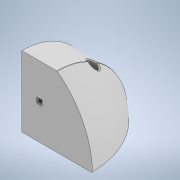
# Autodesk Inventor part: 3DPrintShape
Saved by Autodesk Inventor 2022 (Build 260153000, 153)
## iProperties
Created: 2022-04-20
Part Number: 3DPrintShape
Material: Generic
Document SubType Name: Modeling
Designer: Bruger
Density: 1 g/cm^3
Appearance: Default
Author: Bruger
Autodesk Inventor part; units mm, degrees
ref_plane "YZ Plane" through (0, 0, 0) normal (1, 0, 0) x (0, 1, 0)
ref_plane "XZ Plane" through (0, 0, 0) normal (0, 1, 0) x (-1, 0, 0)
ref_plane "XY Plane" through (0, 0, 0) normal (0, 0, 1) x (1, 0, 0)
sketch "Sketch10" plane through (0, 0, 0) normal (0, 1, 0) x (-1, 0, 0)
  line L0 (0, 0) -> (75, 0)
  line L1 (75, 0) -> (75, -150)
  line L2 (75, -150) -> (0, -150)
  line L3 (0, -150) -> (0, 0)
  line L4 (0, 0) -> (-75, 0)
  line L5 (0, -150) -> (0, 150)
  line L6 (0, 0) -> (-75, 0)
  arc A0 (0, 150) -> (0, -150) centre (112.5, 0) ccw
  dimension "d23" = 75
  dimension "d24" = 150
  dimension "d41" = 300
  dimension "d42" = 75
  constraints: 14 end point, 3 equal length, 3 point on circle, 2 horizontal, 1 centre point, 1 perpendicular, 1 vertical
  measures "d23" distance of L1.end L2.end
  measures "d24" distance of L0.end L1.end
  measures "d41" distance of L2.end L5.end
  measures "d42" distance of L0.start L4.end
revolve "Revolution5" add sketch "Sketch10" angle 90 about axis through (0, 0, 0) along (1, 0, 0) contours L3 A0 L4
sketch "Sketch14" plane through (0, 0, -150) normal (-1, 0, 0) x (0, 0, 1)
  line L0 (0, 0) -> (150, 0) projected
  line L1 (150, 150) -> (150, 0) projected
  arc A0 (150, 150) -> (0, 0) centre (150, 0) ccw
  constraints: 2 point on circle, 1 centre point, 1 coincident
extrude "Extrusion7" add sketch "Sketch14" along normal blind 75
sketch "Sketch15" plane through (-75, 0, -150) normal (-1, 0, 0) x (0, 0, 1)
  line L0 (150, 0) -> (0, 0) projected
  line L1 (75, 0) -> (75, 75)
  line L2 (70, 70) -> (80, 70)
  line L3 (80, 70) -> (80, 80)
  line L4 (80, 80) -> (70, 80)
  line L5 (70, 80) -> (70, 70)
  line L6 (70, 70) -> (80, 80) construction
  line L7 (80, 70) -> (70, 80) construction
  dimension "d46" = 75
  dimension "d47" = 10
  dimension "d48" = 10
  constraints: 14 end point, 3 midpoint, 2 parallel, 1 horizontal, 1 perpendicular, 1 vertical
  measures "d46" distance of L1.start L1.end
  measures "d47" distance of L4.end L3.end
  measures "d48" distance of L3.end L2.end
extrude "Extrusion8" add sketch "Sketch15" along normal blind 10
sketch "Sketch16" plane through (-75, 0, 0) normal (0, 0, 1) x (1, 0, 0)
  line L0 (0, 0) -> (0, 150) projected
  line L1 (0, 75) -> (37.5, 75)
  line L2 (43, 69.5) -> (32, 69.5)
  line L3 (32, 69.5) -> (32, 80.5)
  line L4 (32, 80.5) -> (43, 80.5)
  line L5 (43, 80.5) -> (43, 69.5)
  line L6 (43, 69.5) -> (32, 80.5) construction
  line L7 (32, 69.5) -> (43, 80.5) construction
  point P0 (75, 0)
  dimension "d51" = 37.5
  dimension "d52" = 11
  dimension "d53" = 11
  constraints: 14 end point, 3 midpoint, 2 horizontal, 2 parallel, 1 perpendicular
  measures "d51" distance of L1.start L1.end
  measures "d52" distance of L3.end L4.end
  measures "d53" distance of L2.end L3.end
extrude "Extrusion9" cut sketch "Sketch16" against normal blind 10
sketch "Sketch17" plane through (-75, 0, 0) normal (0, -1, 0) x (1, 0, 0)
  line L0 (0, -150) -> (0, 0) projected
  line L1 (0, -75) -> (75, -75)
  line L2 (75, -150) -> (75, 0) projected
  circle A0 centre (75, -75) radius 6
  circle A1 centre (75, -75) radius 9
  dimension "d56" = 12
  dimension "d57" = 18
  constraints: 2 centre point, 2 coincident, 2 end point, 2 midpoint
  measures "d56" diameter of A0
  measures "d57" diameter of A1
extrude "Extrusion10" cut sketch "Sketch17" against normal blind 197.75
extrude "Extrusion11" add sketch "Sketch17" against normal blind 5 contours A1 L2 A0 L1 | L1 A0 L2 A1 | A1 L2 A0
fillet "Fillet3" radius 2 7 edges at (5.7973, 120.2372, -81.8841) (6.1985, 127.977, -68.4748) (-8.9981, 129.7974, -75.184) (55.2051, 0, -83.8525) (-37.5, 0, -150) (0, 70.3562, -132.4764) (0, 146.1249, -33.8751)
equation "\"shapeMinDepth\" = 7.5"
body "Solid4"
